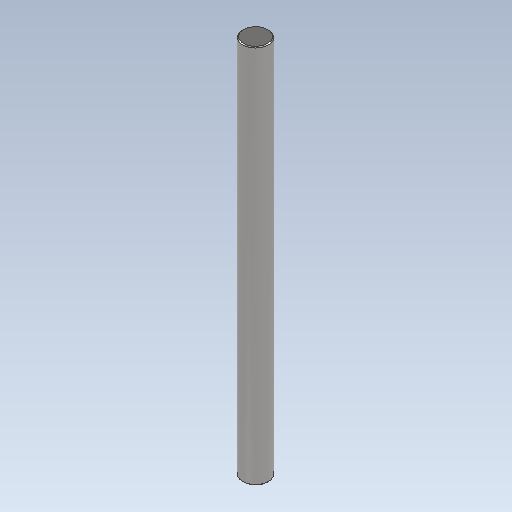
# Autodesk Inventor part: wał_uzębienia
Saved by Autodesk Inventor 2020 (Build 240168000, 168)
## iProperties
Created: 2020-08-10
Part Number: wał_uzębienia
Material: Stainless Steel
Document SubType Name: Modeling
Designer: Hesekiel
Density: 8 g/cm^3
Appearance: Semi-Polished
Mass: 307.753 g
Surface Area: 106.64 cm^2
Volume: 38.4692 cm^3
Author: Hesekiel
Autodesk Inventor part; units mm, degrees
sketch "Sketch1" plane through (0, 0, 0) normal (0, 1, 0) x (-1, 0, 0)
  circle A0 centre (0, 0) radius 7.5
  dimension "d0" = 15
  constraints: 1 centre point, 1 coincident
  measures "d0" diameter of A0
extrude "Extrusion1" add sketch "Sketch1" along normal blind 100
ref_plane "Work Plane1" through (0, 72.5, 0) normal (0, 1, 0) x (1, 0, 0)
sketch "Sketch2" plane through (0, 72.5, 0) normal (0, 1, 0) x (1, 0, 0)
  circle A0 centre (0, 0) radius 7.5 projected
ref_plane "Work Plane2" through (-7.5, 0, 0) normal (1, 0, 0) x (0, 1, 0)
ref_plane "Work Plane3" through (0, 27.5, 0) normal (0, -1, 0) x (1, 0, 0)
sketch "Sketch3" plane through (-7.5, 0, 0) normal (1, 0, 0) x (0, 1, 0)
  line L0 (27.5, -10.5) -> (27.5, 10.5) projected
  line L1 (72.5, 10.5) -> (72.5, -10.5) projected
  line L2 (0, -7.5) -> (0, 7.5) projected
  line L3 (27.5, -3) -> (0, -3)
  line L4 (0, -3) -> (0, 3)
  line L5 (0, 3) -> (27.5, 3)
  line L6 (27.5, 3) -> (27.5, -3)
  line L7 (100, -7.5) -> (100, 7.5) projected
  line L8 (72.5, -3) -> (100, -3)
  line L9 (100, -3) -> (100, 3)
  line L10 (100, 3) -> (72.5, 3)
  line L11 (72.5, 3) -> (72.5, -3)
  line L12 (27.5, -3) -> (72.5, -3)
  line L13 (72.5, -3) -> (72.5, 3)
  line L14 (72.5, 3) -> (27.5, 3)
  line L15 (27.5, 3) -> (27.5, -3)
  point P0 (0, 0)
  constraints: 24 end point, 6 parallel, 5 point on line, 3 horizontal, 3 perpendicular
extrude "Extrusion3" cut sketch "Sketch3" along normal blind 0.5 contours L0 L14 L1 L12 | L1 L10 L7 L8
extrude "Extrusion2" [suppressed]
chamfer "Chamfer1" [suppressed]
sketch "Sketch4" plane through (0, 0, 0) normal (0, -1, 0) x (1, 0, 0)
  circle A0 centre (0, 0) radius 7.5 projected
  circle A1 centre (0, 0) radius 7.5
  constraints: 1 centre point, 1 coincident
extrude "Extrusion4" add sketch "Sketch4" along normal blind 67.5
sketch "Sketch5" plane through (0, 100, 0) normal (0, 1, 0) x (1, 0, 0)
  arc A0 (-7, -2.6926) -> (-7, 2.6926) centre (0, 0) ccw projected
  line L0 (-7, 2.6926) -> (-7, -2.6926) projected
  arc A1 (-7, -2.6926) -> (-7, 2.6926) centre (0, 0) ccw projected
  point P0 (-7, 2.6926)
extrude "Extrusion5" add sketch "Sketch5" along normal blind 52.5
sketch "Sketch6" plane through (-7, 0, 0) normal (-1, 0, 0) x (0, 0, 1)
  line L0 (-2.6926, 27.5) -> (-2.6926, 152.5) projected
  line L1 (2.6926, 152.5) -> (2.6926, 27.5) projected
  line L2 (-2.6926, 152.5) -> (2.6926, 152.5) projected
  line L3 (-2.6926, 152.5) -> (2.6926, 152.5) projected
  line L4 (0, 152.5) -> (0, 72.5)
  line L5 (0, 152.5) -> (80, 152.5) construction
  circle A0 centre (0, 72.5) radius 1.25
  circle A1 centre (0, 72.5) radius 0.75 projected
  circle A2 centre (0, 72.5) radius 0.75
  line L6 (-7.5, -67.5) -> (7.5, -67.5) projected
  line L7 (-2.6926, 26.1771) -> (2.6926, 26.1771)
  line L8 (2.6926, 26.1771) -> (2.6926, -67.5)
  line L9 (2.6926, -67.5) -> (-2.6926, -67.5)
  line L10 (-2.6926, -67.5) -> (-2.6926, 26.1771)
  line L11 (2.6926, 27.5) -> (-2.6926, 27.5) projected
  line L12 (2.6926, 26.1771) -> (2.6926, 27.5)
  line L13 (-2.6926, 27.5) -> (-2.6926, 152.5) projected
  line L14 (-2.6926, 26.1771) -> (-2.6926, 27.5)
  point P0 (0, 0)
  dimension "d23" = 80
  dimension "d24" = 90
  dimension "d25" = 2.5
  dimension "d26" = 1.5
  constraints: 16 end point, 3 vertical, 2 centre point, 2 coincident, 2 horizontal, 2 parallel, 2 perpendicular, 1 midpoint, 1 point on line
  measures "d23" distance of L4.start L4.end
  measures "d24" angle of L4 L5
  measures "d25" diameter of A0
  measures "d26" diameter of A2
extrude "Extrusion6" [suppressed]
chamfer "Chamfer3" [suppressed]
extrude "Extrusion7" cut sketch "Sketch6" along normal blind 0.5 contours L11 L12 L7 L14 | L7 L8 L6 L10
chamfer "Chamfer4" distance 0.5 angle 45 2 edges at (7.5, 152.5, 0) (7.5, -67.5, 0)
body "Solid1"
